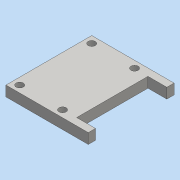
# Autodesk Inventor part: Camera-Holder_Camera-Base
Saved by Autodesk Inventor 2016 SP1 (Build 200210100, 210)
## iProperties
Created: 2016-01-31
Part Number: Camera-Holder_Camera-Base
Material: Generic
Document SubType Name: Modeling
Designer: Mohamed A.
Density: 1 g/cm^3
Appearance: Default
Author: Mohamed A.
Autodesk Inventor part; units mm, degrees
ref_plane "YZ Plane" through (0, 0, 0) normal (1, 0, 0) x (0, 1, 0)
ref_plane "XZ Plane" through (0, 0, 0) normal (0, 1, 0) x (-1, 0, 0)
ref_plane "XY Plane" through (0, 0, 0) normal (0, 0, 1) x (1, 0, 0)
sketch "Sketch1" plane through (0, 0, 0) normal (0, 0, 1) x (1, 0, 0)
  line L0 (-12, 12.5) -> (12, 12.5)
  line L1 (12, -12.5) -> (-12, -12.5)
  line L2 (-12, -12.5) -> (-12, 12.5)
  line L3 (-12, 12.5) -> (12, -12.5) construction
  line L4 (12, 12.5) -> (-12, -12.5) construction
  circle A0 centre (-10, 10.5) radius 1.05
  circle A1 centre (-10, -10.5) radius 1.05
  circle A2 centre (2.5, 10.5) radius 1.05
  circle A3 centre (2.5, -10.5) radius 1.05
  line L5 (12, -10.4) -> (6.5, -10.4)
  line L6 (12, 10.4) -> (6.5, 10.4)
  line L7 (6.5, 10.4) -> (6.5, -10.4)
  line L8 (12, 12.5) -> (12, 10.4)
  line L9 (12, -10.4) -> (12, -12.5)
  point P0 (0, 0)
  dimension "d0" = 24
  dimension "d1" = 25
  dimension "d2" = 2.1
  dimension "d3" = 2
  dimension "d4" = 2
  dimension "d5" = 2.1
  dimension "d6" = 2
  dimension "d7" = 2
  dimension "d8" = 2.1
  dimension "d10" = 2
  dimension "d11" = 2.1
  dimension "d12" = 2
  dimension "d14" = 5.5
  dimension "d16" = 2.1
  dimension "d17" = 2.1
  dimension "d18" = 20.8
  dimension "d19" = 9.5
  dimension "d20" = 9.5
  constraints: 20 end point, 5 perpendicular, 4 centre point, 3 parallel, 2 horizontal, 2 midpoint
  measures "d0" distance of L1.start L1.end
  measures "d1" distance of L0.end L1.start
  measures "d2" diameter of A0
  measures "d3" distance from line of L0 A0.centre
  measures "d4" distance from line of A0.centre L2
  measures "d5" diameter of A1
  measures "d6" distance from line of A1.centre L1
  measures "d7" distance from line of A1.centre L2
  measures "d8" diameter of A2
  measures "d10" distance from line of A2.centre L0
  measures "d11" diameter of A3
  measures "d12" distance from line of L1 A3.centre
  measures "d14" distance of L5.start L5.end
  measures "d16" distance between parallel lines of L1 L5
  measures "d17" distance between parallel lines of L0 L6
  measures "d18" distance of L6.end L5.end
  measures "d19" distance from line of A3.centre L9
  measures "d20" distance from line of A2.centre L8
extrude "Extrusion1" add sketch "Sketch1" along normal blind 3
equation "\"d17\" = d16"
body "Solid1"
